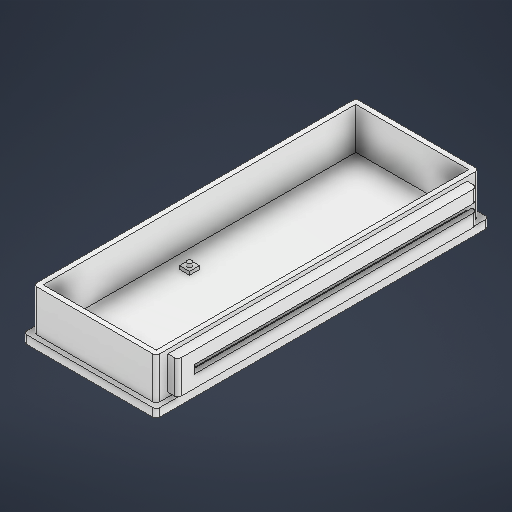
# Autodesk Inventor part: module_command
Saved by Autodesk Inventor 2025.2 (Build 292293000, 293)
## iProperties
Created: 2025-09-05
Part Number: module_command
Material: PC/ABS Plastic
Document SubType Name: Modeling
Designer: sam
Density: 1.1 g/cm^3
Appearance: Smooth - White
Author: sam
Autodesk Inventor part; units mm, degrees
ref_plane "YZ Plane" through (0, 0, 0) normal (1, 0, 0) x (0, 1, 0)
ref_plane "XZ Plane" through (0, 0, 0) normal (0, 1, 0) x (-1, 0, 0)
ref_plane "XY Plane" through (0, 0, 0) normal (0, 0, 1) x (1, 0, 0)
sketch "Sketch1" plane through (0, 0, 0) normal (0, 1, 0) x (-1, 0, 0)
  line L0 (-40, -100) -> (40, -100)
  line L1 (40, -100) -> (40, 100)
  line L2 (40, 100) -> (-40, 100)
  line L3 (-40, 100) -> (-40, -100)
  line L4 (-40, -100) -> (40, 100) construction
  line L5 (40, -100) -> (-40, 100) construction
  point P0 (0, 0)
  dimension "d0" = 80
  dimension "d1" = 200
  constraints: 12 end point, 2 midpoint, 2 parallel, 1 horizontal, 1 perpendicular
  measures "d0" distance of L2.end L1.end
  measures "d1" distance of L1.end L0.end
extrude "Extrusion1" add sketch "Sketch1" along normal blind 5
sketch "Sketch2" plane through (0, 5, 0) normal (0, 1, 0) x (1, 0, 0)
  line L0 (-40, 100) -> (-40, -100) projected
  line L1 (-40, -100) -> (40, -100) projected
  line L2 (40, -100) -> (40, 100) projected
  line L3 (40, 100) -> (-40, 100) projected
  line L4 (37, 97) -> (-37, 97)
  line L5 (-37, 97) -> (-37, -97)
  line L6 (-37, -97) -> (37, -97)
  line L7 (37, -97) -> (37, 97)
  line L8 (37, 97) -> (-37, -97) construction
  line L9 (-37, 97) -> (37, -97) construction
  line L10 (34, 94) -> (-34, 94)
  line L11 (-34, 94) -> (-34, -94)
  line L12 (-34, -94) -> (34, -94)
  line L13 (34, -94) -> (34, 94)
  line L14 (34, 94) -> (-34, -94) construction
  line L15 (-34, 94) -> (34, -94) construction
  point P0 (0, 0)
  dimension "d4" = 3
  dimension "d5" = 3
  dimension "d6" = 3
  dimension "d7" = 3
  constraints: 24 end point, 4 midpoint, 4 parallel, 2 horizontal, 2 perpendicular
  measures "d4" distance between parallel lines of L0 L5
  measures "d5" distance between parallel lines of L1 L6
  measures "d6" distance between parallel lines of L5 L11
  measures "d7" distance between parallel lines of L6 L12
extrude "Extrusion2" add sketch "Sketch2" along normal blind 25 contours L7 L6 L5 L4
fillet "Fillet1" radius 2 4 edges at (-37, 17.5, 97) (37, 17.5, 97) (37, 17.5, -97) (-37, 17.5, -97)
fillet "Fillet2" radius 2 4 edges at (-40, 2.5, 100) (40, 2.5, 100) (40, 2.5, -100) (-40, 2.5, -100)
sketch "Sketch3" plane through (37, 5, 95) normal (1, 0, 0) x (0, 0, -1)
  line L0 (190, 25) -> (190, 0) projected
  line L1 (0, 25) -> (190, 25) projected
  line L2 (0, 0) -> (0, 25) projected
  line L3 (190, 0) -> (0, 0) projected
  line L4 (5, 22.5) -> (185, 22.5)
  line L5 (185, 22.5) -> (185, 2.5)
  line L6 (185, 2.5) -> (5, 2.5)
  line L7 (5, 2.5) -> (5, 22.5)
  line L8 (-2, 25) -> (-2, 0) projected
  line L9 (192, 0) -> (192, 25) projected
  line L10 (195, -5) -> (195, 0) projected
  line L11 (-5, 0) -> (-5, -5) projected
  point P0 (95, -5)
  point P1 (185, 12.5)
  point P2 (-2, 12.5)
  dimension "d33" = 20
  dimension "d34" = 10
  dimension "d35" = 10
  dimension "d36" = 10
  constraints: 8 end point, 2 midpoint, 2 parallel, 1 horizontal, 1 perpendicular
  measures "d33" distance between parallel lines of L4 L6
  measures "d34" distance from line of L4 point (-2, 12.5)
  measures "d35" distance between parallel lines of L10 L5
  measures "d36" distance between parallel lines of L11 L7
extrude "Extrusion3" add sketch "Sketch3" along normal blind 6 contours L4 L5 L6 L7
sketch "Sketch4" plane through (37, 7.5, -90) normal (0, 0, -1) x (-1, 0, 0)
  line L0 (0, 20) -> (0, 0) projected
  line L1 (0, 20) -> (-6, 20) projected
  line L2 (-6, 0) -> (-6, 20) projected
  line L3 (0, 0) -> (-6, 0) projected
  line L4 (-6, 0) -> (-6, 20) projected
  line L5 (-6, 12.5) -> (-3, 12.5)
  line L6 (-3, 12.5) -> (-3, 7.5)
  line L7 (-3, 7.5) -> (-6, 7.5)
  line L8 (-6, 7.5) -> (-6, 12.5)
  line L9 (0, -2.5) -> (0, 22.5) projected
  line L10 (0, 15) -> (-3, 15)
  line L11 (-3, 15) -> (-3, 5)
  line L12 (-3, 5) -> (0, 5)
  line L13 (0, 5) -> (0, 15)
  point P0 (37, -7.5)
  point P1 (-4.5, 12.5)
  point P2 (-6, 7.5)
  point P3 (-3, 7.5)
  point P4 (0, 5)
  point P5 (-3, 12.5)
  point P6 (-1.5, 5)
  dimension "d19" = 3
  dimension "d22" = 5
  dimension "d23" = 5
  dimension "d37" = 2.5
  dimension "d38" = 2.5
  constraints: 16 end point, 4 parallel, 3 point on line, 2 horizontal, 2 midpoint, 2 perpendicular
  measures "d19" distance of L6.end L7.end
  measures "d22" distance between parallel lines of L3 L12
  measures "d23" distance between parallel lines of L1 L10
  measures "d37" distance between parallel lines of L5 L10
  measures "d38" distance from line of point (-1.5, 5) L7
extrude "Extrusion4" cut sketch "Sketch4" against normal blind 170 contours L0 L12 L11 L6 L10 | L5 L6 L7 L2
fillet "Fillet3" radius 2 3 edges at (43, 17.5, 90) (43, 11.25, -90) (43, 23.75, -90)
sketch "Sketch5" plane through (-37, 5, -95) normal (-1, 0, 0) x (0, 0, 1)
  line L0 (0, 25) -> (190, 25) projected
  line L1 (-2, 25) -> (-2, 0) projected
  line L2 (192, 0) -> (192, 25) projected
  line L3 (5, 17.5) -> (175, 17.5)
  line L4 (175, 17.5) -> (175, 7.5)
  line L5 (175, 7.5) -> (5, 7.5)
  line L6 (5, 7.5) -> (5, 17.5)
  line L7 (-5, 0) -> (-5, -5) projected
  line L8 (195, -5) -> (195, 0) projected
  point P0 (95, -5)
  point P1 (192, 12.5)
  dimension "d28" = 10
  dimension "d39" = 10
  dimension "d40" = 20
  dimension "d41" = 5
  constraints: 8 end point, 2 parallel, 1 horizontal, 1 midpoint, 1 perpendicular
  measures "d28" distance of L3.end L4.end
  measures "d39" distance between parallel lines of L7 L6
  measures "d40" distance between parallel lines of L8 L4
  measures "d41" distance from line of point (192, 12.5) L3
extrude "Extrusion5" add sketch "Sketch5" along normal blind 6
sketch "Sketch6" plane through (-37, 12.5, 80) normal (0, 0, 1) x (1, 0, 0)
  line L0 (0, 10) -> (0, 0) projected
  line L1 (0, 10) -> (-6, 10) projected
  line L2 (-6, 0) -> (-6, 10) projected
  line L3 (0, 0) -> (-6, 0) projected
  line L4 (0, 10) -> (-3, 10)
  line L5 (-3, 10) -> (-3, 7.5)
  line L6 (-3, 7.5) -> (0, 7.5)
  line L7 (0, 7.5) -> (0, 10)
  line L8 (0, 0) -> (-3, 0)
  line L9 (-3, 0) -> (-3, 2.5)
  line L10 (-3, 2.5) -> (0, 2.5)
  line L11 (0, 2.5) -> (0, 0)
  point P0 (37, -12.5)
  point P1 (0, 2.5)
  point P2 (-3, 0)
  point P3 (0, 7.5)
  point P4 (-3, 10)
  dimension "d44" = 3
  dimension "d45" = 2.5
  dimension "d46" = 3
  dimension "d47" = 2.5
  constraints: 16 end point, 4 parallel, 2 horizontal, 2 perpendicular
  measures "d44" distance of L6.end L5.end
  measures "d45" distance of L5.end L4.end
  measures "d46" distance of L9.end L10.end
  measures "d47" distance of L8.end L9.end
extrude "Extrusion6" cut sketch "Sketch6" against normal up to surface (170 mm away) contours L0 L6 L5 L1 | L0 L3 L9 L10
fillet "Fillet4" radius 1 18 edges at (-43, 22.5, -5) (-40, 22.5, -5) (-43, 12.5, -5) (-40, 12.5, -5) (-43, 17.5, 80) (-40, 21.25, 80) (-41.5, 22.5, 80) (-41.5, 12.5, 80) (-40, 13.75, 80) (-40, 13.75, -90) (-43, 17.5, -90) (-40, 21.25, -90) (-41.5, 22.5, -90) (-41.5, 12.5, -90) (-38.5, 20, -90) (-38.5, 15, -90) (-38.5, 15, 80) (-38.5, 20, 80)
sketch "Sketch7" plane through (0, 5, 0) normal (0, 1, 0) x (1, 0, 0)
  line L0 (34, 94) -> (-34, 94) projected
  line L1 (-34, 94) -> (-34, -94) projected
  line L2 (-34, -94) -> (34, -94) projected
  line L3 (34, -94) -> (34, 94) projected
  line L4 (25.5, -14.5) -> (-25.5, -14.5)
  line L5 (-25.5, -14.5) -> (-25.5, -85.5)
  line L6 (-25.5, -85.5) -> (25.5, -85.5)
  line L7 (25.5, -85.5) -> (25.5, -14.5)
  line L8 (25.5, -14.5) -> (-25.5, -85.5) construction
  line L9 (-25.5, -14.5) -> (25.5, -85.5) construction
  line L10 (-20, -80) -> (-26, -80)
  line L11 (-26, -80) -> (-26, -86)
  line L12 (-26, -86) -> (-20, -86)
  line L13 (-20, -86) -> (-20, -80)
  line L14 (-20, -80) -> (-26, -86) construction
  line L15 (-26, -80) -> (-20, -86) construction
  line L16 (26, -80) -> (20, -80)
  line L17 (20, -80) -> (20, -86)
  line L18 (20, -86) -> (26, -86)
  line L19 (26, -86) -> (26, -80)
  line L20 (26, -80) -> (20, -86) construction
  line L21 (20, -80) -> (26, -86) construction
  line L22 (26, -14) -> (20, -14)
  line L23 (20, -14) -> (20, -20)
  line L24 (20, -20) -> (26, -20)
  line L25 (26, -20) -> (26, -14)
  line L26 (26, -14) -> (20, -20) construction
  line L27 (20, -14) -> (26, -20) construction
  line L28 (-20, -14) -> (-26, -14)
  line L29 (-26, -14) -> (-26, -20)
  line L30 (-26, -20) -> (-20, -20)
  line L31 (-20, -20) -> (-20, -14)
  line L32 (-20, -14) -> (-26, -20) construction
  line L33 (-26, -14) -> (-20, -20) construction
  point P0 (0, 0)
  point P1 (0, -50)
  point P2 (-23, -83)
  point P3 (16.521, -83.1908)
  point P4 (23, -83)
  point P5 (17.6842, -21.9397)
  point P6 (23, -17)
  point P7 (-22.8956, -21.7602)
  point P8 (-23, -17)
  dimension "d51" = 51
  dimension "d52" = 71
  dimension "d53" = 6
  dimension "d54" = 6
  dimension "d55" = 2.5
  dimension "d56" = 8.5
  dimension "d57" = 2.5
  dimension "d58" = 8.5
  dimension "d59" = 6
  dimension "d60" = 6
  dimension "d61" = 6
  dimension "d62" = 6
  dimension "d63" = 6
  dimension "d64" = 6
  dimension "d65" = 2.5
  dimension "d66" = 2.5
  dimension "d67" = 2.5
  dimension "d68" = 2.5
  dimension "d69" = 2.5
  dimension "d70" = 2.5
  constraints: 60 end point, 10 midpoint, 10 parallel, 5 horizontal, 5 perpendicular
  measures "d51" distance of L6.end L5.end
  measures "d52" distance of L5.end L4.end
  measures "d53" distance of L12.end L11.end
  measures "d54" distance of L11.end L10.end
  measures "d55" distance from line of L6 point (-23, -83)
  measures "d56" distance between parallel lines of L2 L6
  measures "d57" distance from line of point (-23, -83) L5
  measures "d58" distance between parallel lines of L1 L5
  measures "d59" distance of L19.start L17.end
  measures "d60" distance of L17.end L16.end
  measures "d61" distance of L25.start L23.end
  measures "d62" distance of L23.end L22.end
  measures "d63" distance of L31.start L29.end
  measures "d64" distance of L29.end L28.end
  measures "d65" distance from line of L4 point (-23, -17)
  measures "d66" distance from line of L5 point (-23, -17)
  measures "d67" distance from line of L4 point (23, -17)
  measures "d68" distance from line of L7 point (23, -17)
  measures "d69" distance from line of L7 point (23, -83)
  measures "d70" distance from line of L6 point (23, -83)
extrude "Extrusion7" add sketch "Sketch7" along normal blind 4 contours L7 L24 L23 L4 | L4 L23 L22 L25 L24 L7 | L31 L30 L5 L4 | L4 L5 L30 L29 L28 L31 | L16 L19 L18 L17 L6 L7 | L7 L6 L17 L16 | L10 L13 L6 L5 | L5 L6 L13 L12 L11 L10
sketch "Sketch8" plane through (0, 9, 0) normal (0, 1, 0) x (1, 0, 0)
  line L0 (-26, -20) -> (-20, -20) projected
  line L1 (-20, -20) -> (-20, -14) projected
  line L2 (-20, -14) -> (-26, -14) projected
  line L3 (-26, -14) -> (-26, -20) projected
  line L4 (20, -14) -> (20, -20) projected
  line L5 (20, -20) -> (26, -20) projected
  line L6 (26, -20) -> (26, -14) projected
  line L7 (26, -14) -> (20, -14) projected
  line L8 (26, -80) -> (20, -80) projected
  line L9 (20, -80) -> (20, -86) projected
  line L10 (20, -86) -> (26, -86) projected
  line L11 (26, -86) -> (26, -80) projected
  line L12 (-20, -86) -> (-20, -80) projected
  line L13 (-20, -80) -> (-26, -80) projected
  line L14 (-26, -80) -> (-26, -86) projected
  line L15 (-26, -86) -> (-20, -86) projected
  circle A0 centre (-23, -17) radius 1.5
  circle A1 centre (23, -17) radius 1.5
  circle A2 centre (23, -83) radius 1.5
  circle A3 centre (-23, -83) radius 1.5
  point P0 (0, 0)
  dimension "d73" = 3
  dimension "d74" = 3
  dimension "d75" = 3
  dimension "d76" = 3
  constraints: 4 centre point
  measures "d73" diameter of A0
  measures "d74" diameter of A1
  measures "d75" diameter of A2
  measures "d76" diameter of A3
extrude "Extrusion8" cut sketch "Sketch8" against normal blind 2
body "Solid1"
